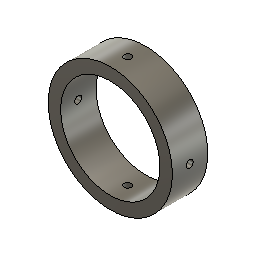
multi-axis test v5 (Autodesk Fusion 360 design; units mm, degrees)
Autodesk Fusion 360 part; units mm, degrees
sketch "Sketch1" plane through (0, 0, 0) normal (0, 0, 1) x (1, 0, 0)
  circle A0 centre (0, 0) radius 14
  circle A1 centre (0, 0) radius 17.5
  dimension "d1" = 35
  dimension "d2" = 28
  constraint coincident A0.centre A1.centre
  measures "d1" diameter of A1
  measures "d2" diameter of A0
extrude "Extrude1" add sketch "Sketch1" along normal blind 10
sketch "Sketch2" plane through (0, 0, 0) normal (0, 1, 0) x (1, 0, 0)
  circle A0 centre (0, -5.08) radius 1
  dimension "d5" = 2
  dimension "d6" = 5.08
  measures "d5" diameter of A0
  measures "d6" distance of origin A0.centre
extrude "Extrude2" cut sketch "Sketch2" along normal through all and the other way through all
sketch "Sketch3" plane through (0, 0, 0) normal (1, 0, 0) x (0, 0, -1)
  circle A0 centre (-5.08, 0) radius 1
  dimension "d9" = 2
  dimension "d10" = 5.08
  measures "d9" diameter of A0
  measures "d10" distance of origin A0.centre
extrude "Extrude3" cut sketch "Sketch3" along normal through all and the other way through all
